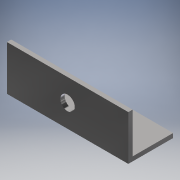
# Autodesk Inventor part: Flywheel top lift wheel bracket
Saved by Autodesk Inventor 2017 (Build 210142000, 142)
## iProperties
Created: 2016-10-25
Part Number: Flywheel top lift wheel bracket
Material: Steel, Alloy
Document SubType Name: Modeling
Designer: Aditya
Density: 7.73 g/cm^3
Appearance: Semi-Polished
Author: Aditya
Autodesk Inventor part; units mm, degrees
ref_plane "YZ Plane" through (0, 0, 0) normal (1, 0, 0) x (0, 1, 0)
ref_plane "XZ Plane" through (0, 0, 0) normal (0, 1, 0) x (-1, 0, 0)
ref_plane "XY Plane" through (0, 0, 0) normal (0, 0, 1) x (1, 0, 0)
sketch "Sketch1" plane through (0, 0, 0) normal (0, 1, 0) x (-1, 0, 0)
  line L0 (0, 0) -> (0, -35.56)
  line L1 (0, -35.56) -> (-106.68, -35.56)
  line L2 (-106.68, -35.56) -> (-106.68, 0)
  line L3 (0, 0) -> (0, 3.81)
  line L4 (0, 3.81) -> (-106.68, 3.81)
  line L5 (-106.68, 3.81) -> (-106.68, 0)
  dimension "d0" = 35.56
  dimension "d1" = 106.68
  dimension "d2" = 3.81
  constraints: 12 end point, 4 perpendicular, 2 vertical
  measures "d0" distance of L0.start L0.end
  measures "d1" distance of L0.end L1.end
  measures "d2" distance of L0.start L3.end
extrude "Extrusion1" add sketch "Sketch1" along normal blind 3.81
sketch "Sketch2" plane through (0, 3.81, 0) normal (0, 1, 0) x (1, 0, 0)
  line L0 (0, 35.56) -> (0, -3.81) projected
  line L1 (0, -3.81) -> (0, 0)
  line L2 (0, 0) -> (106.68, 0)
  line L3 (106.68, -3.81) -> (106.68, 35.56) projected
  line L4 (106.68, -3.81) -> (0, -3.81)
  constraints: 6 end point, 1 parallel, 1 perpendicular, 1 point on line, 1 vertical
extrude "Extrusion2" add sketch "Sketch2" along normal blind 35.56
sketch "Sketch3" plane through (106.68, 3.81, 0) normal (0, 0, -1) x (-1, 0, 0)
  line L0 (106.68, -3.81) -> (106.68, 35.56) projected
  line L1 (106.68, 15.875) -> (0, 15.875)
  line L2 (0, -3.81) -> (0, 35.56) projected
  circle A0 centre (53.34, 15.875) radius 4.7625
  dimension "d10" = 9.525
  constraints: 3 midpoint, 2 end point, 1 centre point
  measures "d10" diameter of A0
extrude "Extrusion3" cut sketch "Sketch3" against normal blind 17.4625
body "Solid1"
